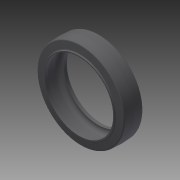
# Autodesk Inventor part: 2.00005.4411 1/4 (T)
Saved by Autodesk Inventor 2014 SP2 (Build 180246200, 246)
## iProperties
Created: 2018-12-09
Part Number: 2.00005.4411 1/4 (T)
Material: Generic
Catalog Web Link: www.cadenas.de
Description: Performa Rubber T-Wheels - Capacity up to 1700 lbs Each
Vendor: COLSONGROUP
Document SubType Name: Modeling
Designer: psadmin
Manufacturer: COLSONGROUP
Mass: 89.8073 g
Surface Area: 339.81 cm^2
Volume: 89.8073 cm^3
Density: 1 g/cm^3
Appearance: PSOLRGB-127-127-127
Category: PARTsolutions
Company: COLSONGROUP
Title: 2.00005.4411 1/4 (T)
Author: Cadenas PARTsolutions
Comments: Wheels - Capacity up to 1700 lbs Each
PSOL_IDENT_0: {$CADENAS_DATA\23d-libs\colsongroup\colson\wheels\performa_rubber\performa_rubber_thread.prj},210 {V
PSOL_IDENT_1: TYP=3D},{NB=2.00005.4411 1/4 (T)},{LINA=2.00005.4411 1/4 (T)},{NN=Performa Rubber T},{DATE=12.06.201
PSOL_IDENT_2: 7 06:51:29},{GEOMDATE=09.06.2017 06:04:53},{VERSION=},{LINEID=10},{WBVAR=WT,SER,D,W,WB,TG},{WBNUMERI
PSOL_IDENT_3: C=D,W}  {NB=2.00005.4411 1/4 (T)},{LINA=2.00005.4411 1/4 (T)},{KT=DUMMY},{PN=2.00005.4411 1/4},{WH=P
PSOL_IDENT_4: erforma Rubber},{WT=PRFG},{SER=2},{SERALG= '1','1 Series (Capacity up to 145 lbs)','2','2 Series (Ca
PSOL_IDENT_5: pacity up to 325 lbs)','3','3 Series (Capacity up to 375 lbs)','4','4 Series (Capacity up to 500 lbs
PSOL_IDENT_6: )','5','5 Series (Capacity up to 675 lbs)' },{D=5},{DALG=2.5,3,3.5,4,5,6},{DPN=05},{W=1.25},{WALG=1.
PSOL_IDENT_7: 25},{WTPN1=4},{WTPN2=4},{WTPN3=},{CAP=320},{CAPALG=320},{CAPPN=},{WB=1},{WBALG= '1','Delrin','5','Ba
PSOL_IDENT_8: ll' },{WBPN=441},{TG=},{TGALG= <'','None'>,' TG1','Metal (TG1)',' TG2','Plastic (TG2)' },{TGPN=},{BB=
PSOL_IDENT_9: 0.50000000},{LBB=0.90625000},{HUB=1.43750000},{SBB=0.37500000},{SBL=1.50000000},{WEIGHT=0.00000000},
PSOL_IDENT_10: {CON=1},{D1=0},{D2=3.88},{BORE=1.19},{ANGS=5},{ANGT=3},{R1=0.25},{TT=0.28},{W1=0.175},{D3=0},{T=0},{
PSOL_IDENT_11: ANGD=5},{ANGU=5},{T2=0.19},{T3=0.06},{R2=0.0625},{W2=1.25},{COLOR=0.50,0.50,0.50,0.00},{TT1=0.28}
NN: Performa Rubber T
NT: Wheels - Capacity up to 1700 lbs Each
NB: 2.00005.4411 1/4 (T)
NBSYN: $PN. (T)
LINA: 2.00005.4411 1/4 (T)
PN: 2.00005.4411 1/4
WH: Performa Rubber
WT: Flat Gray Thread
SER: 2 Series (Capacity up to 325 lbs)
D: 5
W: 0
CAP: 320
WB: Delrin
BB: 0
LBB: 0
HUB: 0
SBB: 0
SBL: 0
WEIGHT: 0
BORE: 1.19
SUPPLIER: COLSONGROUP
ARTICLENO: 2.00005.4411 1/4 (T)
BOMINFO: 2.00005.4411 1/4 (T)
CREATOR: CADENAS GmbH
Autodesk Inventor part; units mm, degrees
sketch "Sketch_8" plane through (0, 0, 0) normal (1, 0, 0) x (0, 1, 0)
  line L0 (0, -15.875) -> (0, 15.875)
  line L1 (49.276, 15.875) -> (49.276, 11.43)
  line L2 (49.276, 11.43) -> (50.038, 11.43)
  arc A0 (56.388, 5.08) -> (50.038, 11.43) centre (50.038, 5.08) ccw
  line L3 (56.388, 5.08) -> (56.388, -5.08)
  arc A1 (50.038, -11.43) -> (56.388, -5.08) centre (50.038, -5.08) ccw
  line L4 (50.038, -11.43) -> (49.276, -11.43)
  line L5 (49.276, -11.43) -> (49.276, -15.875)
  line L6 (49.276, -15.875) -> (50.8, -15.875)
  arc A2 (52.3875, -14.2875) -> (50.8, -15.875) centre (52.3875, -15.875) ccw
  line L7 (52.3875, -14.2875) -> (61.4242, -13.4969)
  arc A3 (61.4242, -13.4969) -> (62.8712, -11.9985) centre (61.2859, -11.9154) ccw
  line L8 (62.8712, -11.9985) -> (63.5, 0)
  line L9 (63.5, 0) -> (62.8712, 11.9985)
  arc A4 (62.8712, 11.9985) -> (61.4242, 13.4969) centre (61.2859, 11.9154) ccw
  line L10 (61.4242, 13.4969) -> (52.3875, 14.2875)
  arc A5 (50.8, 15.875) -> (52.3875, 14.2875) centre (52.3875, 15.875) ccw
  line L11 (50.8, 15.875) -> (49.276, 15.875)
  constraints: 24 end point, 12 point on circle, 6 centre point
revolve "Revolution1" add sketch "Sketch_8" angle 360 about axis through (0, 0, -15.875) along (0, 0, -1)
ref_plane "thread_XY" through (0, 0, 0) normal (0, 0, 1) x (1, 0, 0)
ref_plane "thread_YZ" through (0, 0, 0) normal (1, 0, 0) x (0, 1, 0)
ref_plane "thread_ZX" through (0, 0, 0) normal (0, 1, 0) x (0, 0, 1)
body "Solid1"
